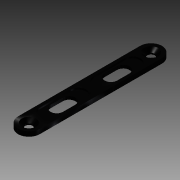
# Autodesk Inventor part: 13_1087_019
Saved by Autodesk Inventor 2014 (Build 180170000, 170)
## iProperties
Created: 2013-09-05
Part Number: 13_1087_019
Material: Allgemein
Document SubType Name: Modeling
Designer: vogel
Density: 1 g/cm^3
Appearance: Schwarz
Author: vogel
Autodesk Inventor part; units mm, degrees
ref_plane "YZ Plane" through (0, 0, 0) normal (1, 0, 0) x (0, 1, 0)
ref_plane "XZ Plane" through (0, 0, 0) normal (0, 1, 0) x (-1, 0, 0)
ref_plane "XY Plane" through (0, 0, 0) normal (0, 0, 1) x (1, 0, 0)
sketch "Skizze1" plane through (0, 0, 0) normal (0, 0, 1) x (1, 0, 0)
  line L0 (-4.9, 0) -> (4.9, 0) projected
  line L1 (0, -32.55) -> (0, 32.55) projected
  line L2 (0, 5) -> (0, -5) construction
  line L3 (0, 19.75) -> (0, -19.75) construction
  line L4 (-3.5, 19.75) -> (-3.5, -19.75)
  line L5 (3.5, -19.75) -> (3.5, 19.75)
  arc A0 (3.5, 19.75) -> (-3.5, 19.75) centre (0, 19.75) ccw
  arc A1 (-3.5, -19.75) -> (3.5, -19.75) centre (0, -19.75) ccw
  line L6 (0, 3.75) -> (0, 13.75) construction
  line L7 (2.5, 3.75) -> (2.5, 13.75)
  line L8 (-2.5, 13.75) -> (-2.5, 3.75)
  arc A2 (-2.5, 3.75) -> (2.5, 3.75) centre (0, 3.75) ccw
  arc A3 (2.5, 13.75) -> (-2.5, 13.75) centre (0, 13.75) ccw
  line L9 (0, -13.75) -> (0, -3.75) construction
  line L10 (2.5, -13.75) -> (2.5, -3.75)
  line L11 (-2.5, -3.75) -> (-2.5, -13.75)
  arc A4 (-2.5, -13.75) -> (2.5, -13.75) centre (0, -13.75) ccw
  arc A5 (2.5, -3.75) -> (-2.5, -3.75) centre (0, -3.75) ccw
  point P0 (0, 0)
  point P1 (0, 0)
  point P2 (0, 0)
  point P3 (0, 8.75)
  point P4 (0, -8.75)
  dimension "d2" = 7
  dimension "d3" = 1.25
  dimension "d4" = 1.25
  dimension "d5" = 23.25
  dimension "d17" = 10
  dimension "d18" = 10
  dimension "d19" = 5
  constraints: 28 end point, 12 point on circle, 12 tangent, 8 point on line, 6 centre point, 4 midpoint, 3 parallel, 1 equal radius, 1 other
  measures "d2" distance between parallel lines of L5 L4
  measures "d3" distance edge to line of A5 L0
  measures "d4" distance edge to line of A2 L0
  measures "d17" distance of L9.start L9.end
  measures "d18" distance of L6.end L6.start
  measures "d19" distance between parallel lines of L7 L8
extrude "Extrusion3" add sketch "Skizze1" along normal blind 0.5 contours L4 A0 L1 A3 L8 A2 L0 | L0 L1 A5 L11 A4 A1 L4 | L1 A2 L7 A3 A0 L5 L0 | L0 L5 A1 L1 A4 L10 A5
sketch "Skizze4" plane through (0, 0, 0) normal (0, 0, -1) x (-1, 0, 0)
  line L0 (3.5, 19.75) -> (3.5, -19.75) projected
  arc A0 (3.5, 19.75) -> (-3.5, 19.75) centre (0, 19.75) ccw projected
  line L1 (-3.5, -19.75) -> (-3.5, 19.75) projected
  arc A1 (-3.5, -19.75) -> (3.5, -19.75) centre (0, -19.75) ccw projected
  point P0 (0, 0)
extrude "Extrusion4" add sketch "Skizze4" along normal blind 1
sketch "Skizze5" plane through (0, 0, 0.5) normal (0, 0, 1) x (1, 0, 0)
  arc A0 (-3.5, -19.75) -> (3.5, -19.75) centre (0, -19.75) ccw projected
  arc A1 (3.5, 19.75) -> (-3.5, 19.75) centre (0, 19.75) ccw projected
  point P0 (0, 0)
  constraints: 2 coincident
hole "Bohrung2" at (0, 19.75, 0.5) at (0, -19.75, 0.5) direction (0, 0, -1) diameter 2.4 end through all countersink diameter 4.6 countersink angle 90
sketch "Skizze6" plane through (0, 0, 0) normal (0, 0, 1) x (1, 0, 0)
  arc A0 (-2.5, -13.75) -> (2.5, -13.75) centre (0, -13.75) ccw projected
  arc A1 (2.5, -3.75) -> (-2.5, -3.75) centre (0, -3.75) ccw projected
  line L0 (-2.5, -3.75) -> (-2.5, -13.75) projected
  line L1 (0, -3.75) -> (0, -13.75)
  line L2 (0, -13.75) -> (0, -8.75)
  line L3 (0, -8.75) -> (-1.5, -8.75)
  line L4 (0, -6.75) -> (0, -10.75) construction
  line L5 (2, -6.75) -> (2, -10.75)
  line L6 (-2, -10.75) -> (-2, -6.75)
  arc A2 (2, -6.75) -> (-2, -6.75) centre (0, -6.75) ccw
  arc A3 (-2, -10.75) -> (2, -10.75) centre (0, -10.75) ccw
  point P0 (0, 0)
  dimension "d32" = 8
  dimension "d33" = 4
  constraints: 14 end point, 4 point on circle, 4 tangent, 2 centre point, 2 midpoint, 2 parallel, 2 point on line, 1 coincident, 1 perpendicular
  measures "d33" distance between parallel lines of L5 L6
extrude "Extrusion5" cut sketch "Skizze6" against normal through all
pattern_linear "Rechteckige Anordnung1" count 2 spacing 17.5 along (0, 1, 0) of "Extrusion5"
